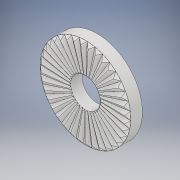
# Autodesk Inventor part: MountRotater
Saved by Autodesk Inventor 2018 (Build 220112000, 112)
## iProperties
Created: 2019-05-28
Part Number: MountRotater
Material: PC/ABS Plastic
Document SubType Name: Modeling
Designer: Ash
Density: 0.357273 g/cm^3
Appearance: Smooth - White
Mass: 0.531337 g
Surface Area: 12.9392 cm^2
Volume: 1.4872 cm^3
Author: Ash
Autodesk Inventor part; units mm, degrees
ref_plane "YZ Plane" through (0, 0, 0) normal (1, 0, 0) x (0, 1, 0)
ref_plane "XZ Plane" through (0, 0, 0) normal (0, 1, 0) x (-1, 0, 0)
sketch "Sketch1" plane through (0, 0, 0) normal (0, 0, 1) x (1, 0, 0)
  circle A0 centre (0, 0) radius 12.446
  line L0 (5.823968, -10.999287) -> (7.63719, -9.827321)
  line L1 (7.63719, -9.827321) -> (2.501569, -3.218949)
  circle A1 centre (0, 0) radius 4.0767
  line L2 (1.907647, -3.602828) -> (5.823968, -10.999287)
  line L3 (2.501569, -3.218949) -> (1.907647, -3.602828)
  line L4 (9.227661, -8.351838) -> (3.02253, -2.735653)
  line L5 (2.50429, -3.216833) -> (7.645495, -9.820862)
  line L6 (7.645495, -9.820862) -> (9.227661, -8.351838)
  line L7 (3.02253, -2.735653) -> (2.50429, -3.216833)
  line L8 (10.537753, -6.622588) -> (3.451652, -2.169236)
  line L9 (3.024841, -2.733097) -> (9.234717, -8.344035)
  line L10 (9.234717, -8.344035) -> (10.537753, -6.622588)
  line L11 (3.451652, -2.169236) -> (3.024841, -2.733097)
  line L12 (11.527661, -4.692115) -> (3.775897, -1.536907)
  line L13 (3.453484, -2.166317) -> (10.543347, -6.613678)
  line L14 (10.543347, -6.613678) -> (11.527661, -4.692115)
  line L15 (3.775897, -1.536907) -> (3.453484, -2.166317)
  line L16 (12.167307, -2.619074) -> (3.985414, -0.85788)
  line L17 (3.777195, -1.533715) -> (11.531623, -4.682369)
  line L18 (11.531623, -4.682369) -> (12.167307, -2.619074)
  line L19 (3.985414, -0.85788) -> (3.777195, -1.533715)
  line L20 (12.437256, -0.466453) -> (4.073836, -0.152787)
  line L21 (3.986138, -0.854511) -> (12.169517, -2.608788)
  line L22 (12.169517, -2.608788) -> (12.437256, -0.466453)
  line L23 (4.073836, -0.152787) -> (3.986138, -0.854511)
  line L24 (12.329305, 1.70034) -> (4.038476, 0.556948)
  line L25 (4.073964, -0.149344) -> (12.437646, -0.45594)
  line L26 (12.437646, -0.45594) -> (12.329305, 1.70034)
  line L27 (4.038476, 0.556948) -> (4.073964, -0.149344)
  line L28 (11.846734, 3.81547) -> (3.88041, 1.249761)
  line L29 (4.038004, 0.560362) -> (12.327863, 1.710762)
  line L30 (12.327863, 1.710762) -> (11.846734, 3.81547)
  line L31 (3.88041, 1.249761) -> (4.038004, 0.560362)
  line L32 (11.004206, 5.814668) -> (3.604439, 1.9046)
  line L33 (3.879352, 1.253041) -> (11.843505, 3.825482)
  line L34 (11.843505, 3.825482) -> (11.004206, 5.814668)
  line L35 (3.604439, 1.9046) -> (3.879352, 1.253041)
  line L36 (9.827321, 7.63719) -> (3.218949, 2.501569)
  line L37 (3.602828, 1.907647) -> (10.999287, 5.823968)
  line L38 (10.999287, 5.823968) -> (9.827321, 7.63719)
  line L39 (3.218949, 2.501569) -> (3.602828, 1.907647)
  line L40 (8.351838, 9.227661) -> (2.735653, 3.02253)
  line L41 (3.216833, 2.50429) -> (9.820862, 7.645495)
  line L42 (9.820862, 7.645495) -> (8.351838, 9.227661)
  line L43 (2.735653, 3.02253) -> (3.216833, 2.50429)
  line L44 (6.622588, 10.537753) -> (2.169236, 3.451652)
  line L45 (2.733097, 3.024841) -> (8.344035, 9.234717)
  line L46 (8.344035, 9.234717) -> (6.622588, 10.537753)
  line L47 (2.169236, 3.451652) -> (2.733097, 3.024841)
  line L48 (4.692115, 11.527661) -> (1.536907, 3.775897)
  line L49 (2.166317, 3.453484) -> (6.613678, 10.543347)
  line L50 (6.613678, 10.543347) -> (4.692115, 11.527661)
  line L51 (1.536907, 3.775897) -> (2.166317, 3.453484)
  line L52 (2.619074, 12.167307) -> (0.85788, 3.985414)
  line L53 (1.533715, 3.777195) -> (4.682369, 11.531623)
  line L54 (4.682369, 11.531623) -> (2.619074, 12.167307)
  line L55 (0.85788, 3.985414) -> (1.533715, 3.777195)
  line L56 (0.466453, 12.437256) -> (0.152787, 4.073836)
  line L57 (0.854511, 3.986138) -> (2.608788, 12.169517)
  line L58 (2.608788, 12.169517) -> (0.466453, 12.437256)
  line L59 (0.152787, 4.073836) -> (0.854511, 3.986138)
  line L60 (-1.70034, 12.329305) -> (-0.556948, 4.038476)
  line L61 (0.149344, 4.073964) -> (0.45594, 12.437646)
  line L62 (0.45594, 12.437646) -> (-1.70034, 12.329305)
  line L63 (-0.556948, 4.038476) -> (0.149344, 4.073964)
  line L64 (-3.81547, 11.846734) -> (-1.249761, 3.88041)
  line L65 (-0.560362, 4.038004) -> (-1.710762, 12.327863)
  line L66 (-1.710762, 12.327863) -> (-3.81547, 11.846734)
  line L67 (-1.249761, 3.88041) -> (-0.560362, 4.038004)
  line L68 (-5.814668, 11.004206) -> (-1.9046, 3.604439)
  line L69 (-1.253041, 3.879352) -> (-3.825482, 11.843505)
  line L70 (-3.825482, 11.843505) -> (-5.814668, 11.004206)
  line L71 (-1.9046, 3.604439) -> (-1.253041, 3.879352)
  line L72 (-7.63719, 9.827321) -> (-2.501569, 3.218949)
  line L73 (-1.907647, 3.602828) -> (-5.823968, 10.999287)
  line L74 (-5.823968, 10.999287) -> (-7.63719, 9.827321)
  line L75 (-2.501569, 3.218949) -> (-1.907647, 3.602828)
  line L76 (-9.227661, 8.351838) -> (-3.02253, 2.735653)
  line L77 (-2.50429, 3.216833) -> (-7.645495, 9.820862)
  line L78 (-7.645495, 9.820862) -> (-9.227661, 8.351838)
  line L79 (-3.02253, 2.735653) -> (-2.50429, 3.216833)
  line L80 (-10.537753, 6.622588) -> (-3.451652, 2.169236)
  line L81 (-3.024841, 2.733097) -> (-9.234717, 8.344035)
  line L82 (-9.234717, 8.344035) -> (-10.537753, 6.622588)
  line L83 (-3.451652, 2.169236) -> (-3.024841, 2.733097)
  line L84 (-11.527661, 4.692115) -> (-3.775897, 1.536907)
  line L85 (-3.453484, 2.166317) -> (-10.543347, 6.613678)
  line L86 (-10.543347, 6.613678) -> (-11.527661, 4.692115)
  line L87 (-3.775897, 1.536907) -> (-3.453484, 2.166317)
  line L88 (-12.167307, 2.619074) -> (-3.985414, 0.85788)
  line L89 (-3.777195, 1.533715) -> (-11.531623, 4.682369)
  line L90 (-11.531623, 4.682369) -> (-12.167307, 2.619074)
  line L91 (-3.985414, 0.85788) -> (-3.777195, 1.533715)
  line L92 (-12.437256, 0.466453) -> (-4.073836, 0.152787)
  line L93 (-3.986138, 0.854511) -> (-12.169517, 2.608788)
  line L94 (-12.169517, 2.608788) -> (-12.437256, 0.466453)
  line L95 (-4.073836, 0.152787) -> (-3.986138, 0.854511)
  line L96 (-12.329305, -1.70034) -> (-4.038476, -0.556948)
  line L97 (-4.073964, 0.149344) -> (-12.437646, 0.45594)
  line L98 (-12.437646, 0.45594) -> (-12.329305, -1.70034)
  line L99 (-4.038476, -0.556948) -> (-4.073964, 0.149344)
  line L100 (-11.846734, -3.81547) -> (-3.88041, -1.249761)
  line L101 (-4.038004, -0.560362) -> (-12.327863, -1.710762)
  line L102 (-12.327863, -1.710762) -> (-11.846734, -3.81547)
  line L103 (-3.88041, -1.249761) -> (-4.038004, -0.560362)
  line L104 (-11.004206, -5.814668) -> (-3.604439, -1.9046)
  line L105 (-3.879352, -1.253041) -> (-11.843505, -3.825482)
  line L106 (-11.843505, -3.825482) -> (-11.004206, -5.814668)
  line L107 (-3.604439, -1.9046) -> (-3.879352, -1.253041)
  line L108 (-9.827321, -7.63719) -> (-3.218949, -2.501569)
  line L109 (-3.602828, -1.907647) -> (-10.999287, -5.823968)
  line L110 (-10.999287, -5.823968) -> (-9.827321, -7.63719)
  line L111 (-3.218949, -2.501569) -> (-3.602828, -1.907647)
  line L112 (-8.351838, -9.227661) -> (-2.735653, -3.02253)
  line L113 (-3.216833, -2.50429) -> (-9.820862, -7.645495)
  line L114 (-9.820862, -7.645495) -> (-8.351838, -9.227661)
  line L115 (-2.735653, -3.02253) -> (-3.216833, -2.50429)
  line L116 (-6.622588, -10.537753) -> (-2.169236, -3.451652)
  line L117 (-2.733097, -3.024841) -> (-8.344035, -9.234717)
  line L118 (-8.344035, -9.234717) -> (-6.622588, -10.537753)
  line L119 (-2.169236, -3.451652) -> (-2.733097, -3.024841)
  line L120 (-4.692115, -11.527661) -> (-1.536907, -3.775897)
  line L121 (-2.166317, -3.453484) -> (-6.613678, -10.543347)
  line L122 (-6.613678, -10.543347) -> (-4.692115, -11.527661)
  line L123 (-1.536907, -3.775897) -> (-2.166317, -3.453484)
  line L124 (-2.619074, -12.167307) -> (-0.85788, -3.985414)
  line L125 (-1.533715, -3.777195) -> (-4.682369, -11.531623)
  line L126 (-4.682369, -11.531623) -> (-2.619074, -12.167307)
  line L127 (-0.85788, -3.985414) -> (-1.533715, -3.777195)
  line L128 (-0.466453, -12.437256) -> (-0.152787, -4.073836)
  line L129 (-0.854511, -3.986138) -> (-2.608788, -12.169517)
  line L130 (-2.608788, -12.169517) -> (-0.466453, -12.437256)
  line L131 (-0.152787, -4.073836) -> (-0.854511, -3.986138)
  line L132 (1.70034, -12.329305) -> (0.556948, -4.038476)
  line L133 (-0.149344, -4.073964) -> (-0.45594, -12.437646)
  line L134 (-0.45594, -12.437646) -> (1.70034, -12.329305)
  line L135 (0.556948, -4.038476) -> (-0.149344, -4.073964)
  line L136 (3.81547, -11.846734) -> (1.249761, -3.88041)
  line L137 (0.560362, -4.038004) -> (1.710762, -12.327863)
  line L138 (1.710762, -12.327863) -> (3.81547, -11.846734)
  line L139 (1.249761, -3.88041) -> (0.560362, -4.038004)
  line L140 (5.814668, -11.004206) -> (1.9046, -3.604439)
  line L141 (1.253041, -3.879352) -> (3.825482, -11.843505)
  line L142 (3.825482, -11.843505) -> (5.814668, -11.004206)
  line L143 (1.9046, -3.604439) -> (1.253041, -3.879352)
  dimension "d0" = 24.892
  dimension "d1" = 2.159
  dimension "d12" = 8.1534
  dimension "d23" = 360
  constraints: 288 end point, 4 point on circle, 2 centre point, 2 coincident, 290 other
  measures "d0" diameter of A0
  measures "d1" distance of L0.start L0.end
  measures "d12" diameter of A1
ref_plane "Work Plane1" through (0, 0, 0.9144) normal (0, 0, 1) x (1, 0, 0)
sketch "Sketch1 outline for Extrusion1" plane through (0, 0, 0) normal (0, 0, 1) x (1, 0, 0)
  line L0 (1.907647, -3.602828) -> (5.823968, -10.999287)
  arc A0 (2.501569, -3.218949) -> (1.907647, -3.602828) centre (0, 0) cw
  line L1 (7.63719, -9.827321) -> (2.501569, -3.218949)
  line L2 (5.823968, -10.999287) -> (7.63719, -9.827321)
  line L3 (5.814668, -11.004206) -> (3.825482, -11.843505)
  line L4 (3.825482, -11.843505) -> (1.253041, -3.879352)
  line L5 (1.253041, -3.879352) -> (1.9046, -3.604439)
  line L6 (1.9046, -3.604439) -> (5.814668, -11.004206)
  line L7 (3.81547, -11.846734) -> (1.710762, -12.327863)
  line L8 (1.710762, -12.327863) -> (0.560362, -4.038004)
  line L9 (0.560362, -4.038004) -> (1.249761, -3.88041)
  line L10 (1.249761, -3.88041) -> (3.81547, -11.846734)
  line L11 (1.70034, -12.329305) -> (-0.45594, -12.437646)
  line L12 (-0.45594, -12.437646) -> (-0.149344, -4.073964)
  line L13 (-0.149344, -4.073964) -> (0.556948, -4.038476)
  line L14 (0.556948, -4.038476) -> (1.70034, -12.329305)
  line L15 (-0.466453, -12.437256) -> (-2.608788, -12.169517)
  line L16 (-2.608788, -12.169517) -> (-0.854511, -3.986138)
  line L17 (-0.854511, -3.986138) -> (-0.152787, -4.073836)
  line L18 (-0.152787, -4.073836) -> (-0.466453, -12.437256)
  line L19 (-2.619074, -12.167307) -> (-4.682369, -11.531623)
  line L20 (-4.682369, -11.531623) -> (-1.533715, -3.777195)
  line L21 (-1.533715, -3.777195) -> (-0.85788, -3.985414)
  line L22 (-0.85788, -3.985414) -> (-2.619074, -12.167307)
  line L23 (-4.692115, -11.527661) -> (-6.613678, -10.543347)
  line L24 (-6.613678, -10.543347) -> (-2.166317, -3.453484)
  line L25 (-2.166317, -3.453484) -> (-1.536907, -3.775897)
  line L26 (-1.536907, -3.775897) -> (-4.692115, -11.527661)
  line L27 (-6.622588, -10.537753) -> (-8.344035, -9.234717)
  line L28 (-8.344035, -9.234717) -> (-2.733097, -3.024841)
  line L29 (-2.733097, -3.024841) -> (-2.169236, -3.451652)
  line L30 (-2.169236, -3.451652) -> (-6.622588, -10.537753)
  line L31 (-8.351838, -9.227661) -> (-9.820862, -7.645495)
  line L32 (-9.820862, -7.645495) -> (-3.216833, -2.50429)
  line L33 (-3.216833, -2.50429) -> (-2.735653, -3.02253)
  line L34 (-2.735653, -3.02253) -> (-8.351838, -9.227661)
  line L35 (-9.827321, -7.63719) -> (-10.999287, -5.823968)
  line L36 (-10.999287, -5.823968) -> (-3.602828, -1.907647)
  line L37 (-3.602828, -1.907647) -> (-3.218949, -2.501569)
  line L38 (-3.218949, -2.501569) -> (-9.827321, -7.63719)
  line L39 (-11.004206, -5.814668) -> (-11.843505, -3.825482)
  line L40 (-11.843505, -3.825482) -> (-3.879352, -1.253041)
  line L41 (-3.879352, -1.253041) -> (-3.604439, -1.9046)
  line L42 (-3.604439, -1.9046) -> (-11.004206, -5.814668)
  line L43 (-11.846734, -3.81547) -> (-12.327863, -1.710762)
  line L44 (-12.327863, -1.710762) -> (-4.038004, -0.560362)
  line L45 (-4.038004, -0.560362) -> (-3.88041, -1.249761)
  line L46 (-3.88041, -1.249761) -> (-11.846734, -3.81547)
  line L47 (-12.329305, -1.70034) -> (-12.437646, 0.45594)
  line L48 (-12.437646, 0.45594) -> (-4.073964, 0.149344)
  line L49 (-4.073964, 0.149344) -> (-4.038476, -0.556948)
  line L50 (-4.038476, -0.556948) -> (-12.329305, -1.70034)
  line L51 (-12.437256, 0.466453) -> (-12.169517, 2.608788)
  line L52 (-12.169517, 2.608788) -> (-3.986138, 0.854511)
  line L53 (-3.986138, 0.854511) -> (-4.073836, 0.152787)
  line L54 (-4.073836, 0.152787) -> (-12.437256, 0.466453)
  line L55 (-12.167307, 2.619074) -> (-11.531623, 4.682369)
  line L56 (-11.531623, 4.682369) -> (-3.777195, 1.533715)
  line L57 (-3.777195, 1.533715) -> (-3.985414, 0.85788)
  line L58 (-3.985414, 0.85788) -> (-12.167307, 2.619074)
  line L59 (-11.527661, 4.692115) -> (-10.543347, 6.613678)
  line L60 (-10.543347, 6.613678) -> (-3.453484, 2.166317)
  line L61 (-3.453484, 2.166317) -> (-3.775897, 1.536907)
  line L62 (-3.775897, 1.536907) -> (-11.527661, 4.692115)
  line L63 (-10.537753, 6.622588) -> (-9.234717, 8.344035)
  line L64 (-9.234717, 8.344035) -> (-3.024841, 2.733097)
  line L65 (-3.024841, 2.733097) -> (-3.451652, 2.169236)
  line L66 (-3.451652, 2.169236) -> (-10.537753, 6.622588)
  line L67 (-9.227661, 8.351838) -> (-7.645495, 9.820862)
  line L68 (-7.645495, 9.820862) -> (-2.50429, 3.216833)
  line L69 (-2.50429, 3.216833) -> (-3.02253, 2.735653)
  line L70 (-3.02253, 2.735653) -> (-9.227661, 8.351838)
  line L71 (-7.63719, 9.827321) -> (-5.823968, 10.999287)
  line L72 (-5.823968, 10.999287) -> (-1.907647, 3.602828)
  line L73 (-1.907647, 3.602828) -> (-2.501569, 3.218949)
  line L74 (-2.501569, 3.218949) -> (-7.63719, 9.827321)
  line L75 (-5.814668, 11.004206) -> (-3.825482, 11.843505)
  line L76 (-3.825482, 11.843505) -> (-1.253041, 3.879352)
  line L77 (-1.253041, 3.879352) -> (-1.9046, 3.604439)
  line L78 (-1.9046, 3.604439) -> (-5.814668, 11.004206)
  line L79 (-3.81547, 11.846734) -> (-1.710762, 12.327863)
  line L80 (-1.710762, 12.327863) -> (-0.560362, 4.038004)
  line L81 (-0.560362, 4.038004) -> (-1.249761, 3.88041)
  line L82 (-1.249761, 3.88041) -> (-3.81547, 11.846734)
  line L83 (-1.70034, 12.329305) -> (0.45594, 12.437646)
  line L84 (0.45594, 12.437646) -> (0.149344, 4.073964)
  line L85 (0.149344, 4.073964) -> (-0.556948, 4.038476)
  line L86 (-0.556948, 4.038476) -> (-1.70034, 12.329305)
  line L87 (0.466453, 12.437256) -> (2.608788, 12.169517)
  line L88 (2.608788, 12.169517) -> (0.854511, 3.986138)
  line L89 (0.854511, 3.986138) -> (0.152787, 4.073836)
  line L90 (0.152787, 4.073836) -> (0.466453, 12.437256)
  line L91 (2.619074, 12.167307) -> (4.682369, 11.531623)
  line L92 (4.682369, 11.531623) -> (1.533715, 3.777195)
  line L93 (1.533715, 3.777195) -> (0.85788, 3.985414)
  line L94 (0.85788, 3.985414) -> (2.619074, 12.167307)
  line L95 (4.692115, 11.527661) -> (6.613678, 10.543347)
  line L96 (6.613678, 10.543347) -> (2.166317, 3.453484)
  line L97 (2.166317, 3.453484) -> (1.536907, 3.775897)
  line L98 (1.536907, 3.775897) -> (4.692115, 11.527661)
  line L99 (6.622588, 10.537753) -> (8.344035, 9.234717)
  line L100 (8.344035, 9.234717) -> (2.733097, 3.024841)
  line L101 (2.733097, 3.024841) -> (2.169236, 3.451652)
  line L102 (2.169236, 3.451652) -> (6.622588, 10.537753)
  line L103 (8.351838, 9.227661) -> (9.820862, 7.645495)
  line L104 (9.820862, 7.645495) -> (3.216833, 2.50429)
  line L105 (3.216833, 2.50429) -> (2.735653, 3.02253)
  line L106 (2.735653, 3.02253) -> (8.351838, 9.227661)
  line L107 (9.827321, 7.63719) -> (10.999287, 5.823968)
  line L108 (10.999287, 5.823968) -> (3.602828, 1.907647)
  line L109 (3.602828, 1.907647) -> (3.218949, 2.501569)
  line L110 (3.218949, 2.501569) -> (9.827321, 7.63719)
  line L111 (11.004206, 5.814668) -> (11.843505, 3.825482)
  line L112 (11.843505, 3.825482) -> (3.879352, 1.253041)
  line L113 (3.879352, 1.253041) -> (3.604439, 1.9046)
  line L114 (3.604439, 1.9046) -> (11.004206, 5.814668)
  line L115 (11.846734, 3.81547) -> (12.327863, 1.710762)
  line L116 (12.327863, 1.710762) -> (4.038004, 0.560362)
  line L117 (4.038004, 0.560362) -> (3.88041, 1.249761)
  line L118 (3.88041, 1.249761) -> (11.846734, 3.81547)
  line L119 (12.329305, 1.70034) -> (12.437646, -0.45594)
  line L120 (12.437646, -0.45594) -> (4.073964, -0.149344)
  line L121 (4.073964, -0.149344) -> (4.038476, 0.556948)
  line L122 (4.038476, 0.556948) -> (12.329305, 1.70034)
  line L123 (12.437256, -0.466453) -> (12.169517, -2.608788)
  line L124 (12.169517, -2.608788) -> (3.986138, -0.854511)
  line L125 (3.986138, -0.854511) -> (4.073836, -0.152787)
  line L126 (4.073836, -0.152787) -> (12.437256, -0.466453)
  line L127 (12.167307, -2.619074) -> (11.531623, -4.682369)
  line L128 (11.531623, -4.682369) -> (3.777195, -1.533715)
  line L129 (3.777195, -1.533715) -> (3.985414, -0.85788)
  line L130 (3.985414, -0.85788) -> (12.167307, -2.619074)
  line L131 (11.527661, -4.692115) -> (10.543347, -6.613678)
  line L132 (10.543347, -6.613678) -> (3.453484, -2.166317)
  line L133 (3.453484, -2.166317) -> (3.775897, -1.536907)
  line L134 (3.775897, -1.536907) -> (11.527661, -4.692115)
  line L135 (10.537753, -6.622588) -> (9.234717, -8.344035)
  line L136 (9.234717, -8.344035) -> (3.024841, -2.733097)
  line L137 (3.024841, -2.733097) -> (3.451652, -2.169236)
  line L138 (3.451652, -2.169236) -> (10.537753, -6.622588)
  line L139 (9.227661, -8.351838) -> (7.645495, -9.820862)
  line L140 (7.645495, -9.820862) -> (2.50429, -3.216833)
  line L141 (2.50429, -3.216833) -> (3.02253, -2.735653)
  line L142 (3.02253, -2.735653) -> (9.227661, -8.351838)
extrude "Extrusion1" add sketch "Sketch1 outline for Extrusion1" along normal blind 25.4 draft -55
sketch "Sketch3" plane through (0, 0, 0) normal (0, 0, 1) x (1, 0, 0)
  line L0 (-1.70034, 12.329305) -> (0.45594, 12.437646)
  circle A0 centre (0, 0) radius 12.446
  circle A1 centre (0, 0) radius 4.061337
  constraints: 2 coincident, 1 centre point, 3 other
extrude "Extrusion3" add sketch "Sketch3" against normal blind 3.175
body "Solid1"
